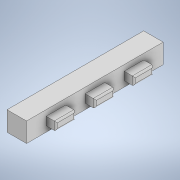
# Autodesk Inventor part: WeaponMountTenonTest
Saved by Autodesk Inventor 2020 (Build 240168000, 168)
## iProperties
Created: 2024-02-07
Part Number: WeaponMountTenonTest
Material: Generic
Document SubType Name: Modeling
Designer: smz3rm
Density: 1 g/cm^3
Appearance: Default
Author: smz3rm
Autodesk Inventor part; units mm, degrees
ref_plane "YZ Plane" through (0, 0, 0) normal (1, 0, 0) x (0, 1, 0)
ref_plane "XZ Plane" through (0, 0, 0) normal (0, 1, 0) x (-1, 0, 0)
ref_plane "XY Plane" through (0, 0, 0) normal (0, 0, 1) x (1, 0, 0)
sketch "Sketch1" plane through (0, 0, 0) normal (1, 0, 0) x (0, 1, 0)
  line L0 (3, 21) -> (-3, 21)
  line L1 (-3, 21) -> (-3, -21)
  line L2 (-3, -21) -> (3, -21)
  line L3 (3, -21) -> (3, 21)
  line L4 (3, 21) -> (-3, -21) construction
  line L5 (-3, 21) -> (3, -21) construction
  point P0 (0, 0)
  dimension "d0" = 6
  dimension "d1" = 42
  constraints: 12 end point, 2 midpoint, 2 parallel, 1 horizontal, 1 perpendicular
  measures "d0" distance of L2.end L1.end
  measures "d1" distance of L1.end L0.end
extrude "Extrusion1" add sketch "Sketch1" along normal blind 6
sketch "Sketch2" plane through (6, 0, 0) normal (1, 0, 0) x (0, 0, -1)
  line L0 (-15, 1.25) -> (-9, 1.25)
  line L1 (-9, 1.25) -> (-9, -1.25)
  line L2 (-9, -1.25) -> (-15, -1.25)
  line L3 (-15, -1.25) -> (-15, 1.25)
  line L4 (-15, 1.25) -> (-9, -1.25) construction
  line L5 (-9, 1.25) -> (-15, -1.25) construction
  line L6 (-21, 3) -> (-21, -3) projected
  line L7 (29.4, 0) -> (-29.4, 0) projected
  line L8 (-3, 1.25) -> (3, 1.25)
  line L9 (-3, -1.25) -> (-3, 1.25)
  line L10 (3, -1.25) -> (-3, -1.25)
  line L11 (3, 1.25) -> (3, -1.25)
  line L12 (9, 1.25) -> (15, 1.25)
  line L13 (9, -1.25) -> (9, 1.25)
  line L14 (15, -1.25) -> (9, -1.25)
  line L15 (15, 1.25) -> (15, -1.25)
  point P0 (0, 0)
  point P1 (-12, 0)
  point P2 (-12, 0)
  dimension "d4" = 6
  dimension "d5" = 2.5
  dimension "d6" = 6
  dimension "d9" = 12
  constraints: 28 end point, 3 midpoint, 2 horizontal, 2 parallel, 1 perpendicular, 1 point on line, 16 other
  measures "d4" distance of L1.end L2.end
  measures "d5" distance of L0.end L1.end
  measures "d6" distance between parallel lines of L6 L3
  measures "d9" distance of L0.start L8.start
extrude "Extrusion2" add sketch "Sketch2" along normal blind 3
fillet "Fillet1" radius 0.5 12 edges at (9, 1.25, 12) (9, 0, 15) (9, -1.25, 12) (9, 0, 9) (9, 0, 3) (9, 1.25, 0) (9, -1.25, 0) (9, 0, -3) (9, 0, -9) (9, 1.25, -12) (9, -1.25, -12) (9, 0, -15)
equation "\"d0\" = WeaponMountBaseThickness"
equation "\"d1\" = 7 * SlotWidth"
equation "\"d2\" = WeaponMountBaseThickness"
equation "\"d4\" = SlotWidth"
equation "\"d5\" = SlotHeight"
equation "\"d6\" = SlotWidth"
equation "\"d9\" = 2 * SlotWidth"
equation "\"d14\" = WeaponMountThickness"
equation "\"WeaponMountBaseThickness\" = 6"
equation "\"SlotWidth\" = 6"
equation "\"SlotHeight\" = 2.5"
equation "\"WeaponMountThickness\" = 3"
body "Solid1"
